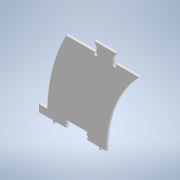
# Autodesk Inventor part: Support C - V2
Saved by Autodesk Inventor 2021 (Build 250183000, 183)
## iProperties
Created: 2020-07-22
Part Number: Support C - V2
Material: Generic
Document SubType Name: Modeling
Designer: Dan Wikman
Density: 1 g/cm^3
Appearance: Default
Author: Dan Wikman
Autodesk Inventor part; units mm, degrees
ref_plane "YZ Plane" through (0, 0, 0) normal (1, 0, 0) x (0, 1, 0)
ref_plane "XZ Plane" through (0, 0, 0) normal (0, 1, 0) x (-1, 0, 0)
ref_plane "XY Plane" through (0, 0, 0) normal (0, 0, 1) x (1, 0, 0)
sketch "Sketch1" plane through (0, 0, 0) normal (0, 0, 1) x (1, 0, 0)
  arc A0 (0, 550) -> (-200, 512.3475) centre (0, 0) ccw construction
  line L0 (-150, -512.4764) -> (-150, -323.4644) construction
  line L1 (-472.3938, -281.6809) -> (-252.3938, -281.6809) construction
  line L2 (-489.0365, 251.6809) -> (-252.3938, 251.6809) construction
  line L3 (-150.0879, 323.2475) -> (-150.0879, 512.2595) construction
  line L4 (-472.3938, 281.6809) -> (-252.3938, 281.6809) construction
  line L5 (-472.3938, -251.6809) -> (-252.3938, -251.6809) construction
  line L6 (-356.435, 15) -> (-576.435, 15) construction
  line L7 (-472.3938, -281.6809) -> (-472.3938, -251.6809) construction
  line L8 (-252.3938, -281.6809) -> (-252.3938, -251.6809) construction
  line L9 (-252.3938, 281.6809) -> (-252.3938, 251.6809) construction
  line L10 (-472.3938, 281.6809) -> (-472.3938, 251.6809) construction
  line L11 (-356.435, 15) -> (-356.435, -15) construction
  line L12 (-356.435, -15) -> (-576.435, -15) construction
  line L13 (-576.435, -15) -> (-576.435, 15) construction
  arc A1 (-0.0879, 356.3469) -> (-150.0879, 323.2475) centre (-0.0879, -0.0881) ccw construction
  arc A2 (-150, -323.4644) -> (-1.4799, -356.5203) centre (-0.0879, -0.0881) ccw construction
  arc A3 (-156.5047, -512.4764) -> (-160, -512.3475) centre (-158.25, -512.3475) ccw construction
  arc A4 (-190, -512.3475) -> (-193.5, -512.3475) centre (-191.75, -512.3475) ccw construction
  line L14 (-178.75, -519.0975) -> (-175, -519.0975) construction
  line L15 (-178.75, -529.0975) -> (-175, -529.0975) construction
  line L16 (-175, -519.0975) -> (-175, -529.0975) construction
  arc A5 (-178.75, -519.0975) -> (-178.75, -522.5975) centre (-178.75, -520.8475) ccw construction
  arc A6 (-178.75, -525.5975) -> (-178.75, -529.0975) centre (-178.75, -527.3475) ccw construction
  line L17 (-171.25, -519.0975) -> (-175, -519.0975) construction
  line L18 (-171.25, -529.0975) -> (-175, -529.0975) construction
  arc A7 (-171.25, -522.5975) -> (-171.25, -519.0975) centre (-171.25, -520.8475) ccw construction
  arc A8 (-171.25, -529.0975) -> (-171.25, -525.5975) centre (-171.25, -527.3475) ccw construction
  line L19 (-252.3938, 251.6809) -> (-489.0365, 251.6809) construction
  arc A9 (-192.6667, 512.3475) -> (-190, 512.3475) centre (-191.3333, 512.3475) ccw construction
  line L20 (-157.3333, 512.3475) -> (-150, 512.3475) construction
  line L21 (-192.6667, 512.3475) -> (-200, 512.3475) construction
  arc A10 (-160, 512.3475) -> (-157.3333, 512.3475) centre (-158.6667, 512.3475) ccw construction
  line L22 (-171.25, 517.8475) -> (-175, 517.8475) construction
  line L23 (-171.25, 520.5142) -> (-171.25, 525.1809) construction
  line L24 (-161.3333, 532.3475) -> (-188.6667, 532.3475) construction
  line L25 (-190, 531.0142) -> (-190, 512.3475) construction
  line L26 (-160, 531.0142) -> (-160, 512.3475) construction
  arc A11 (-160, 531.0142) -> (-161.3333, 532.3475) centre (-161.3333, 531.0142) ccw construction
  arc A12 (-188.6667, 532.3475) -> (-190, 531.0142) centre (-188.6667, 531.0142) ccw construction
  line L27 (-171.25, 527.8475) -> (-175, 527.8475) construction
  line L28 (-175, 532.3475) -> (-175, 535.9358) construction
  line L29 (-175, 517.8475) -> (-175, 527.8475) construction
  arc A13 (-171.25, 517.8475) -> (-171.25, 520.5142) centre (-171.25, 519.1809) ccw construction
  arc A14 (-171.25, 525.1809) -> (-171.25, 527.8475) centre (-171.25, 526.5142) ccw construction
  line L30 (-178.75, 517.8475) -> (-175, 517.8475) construction
  arc A15 (-178.75, 520.5142) -> (-178.75, 517.8475) centre (-178.75, 519.1809) ccw construction
  line L31 (-178.75, 520.5142) -> (-178.75, 525.1809) construction
  arc A16 (-178.75, 527.8475) -> (-178.75, 525.1809) centre (-178.75, 526.5142) ccw construction
  line L32 (-178.75, 527.8475) -> (-175, 527.8475) construction
  arc A17 (-334.9122, -265.623) -> (-335.582, -268.123) centre (-330.582, -268.123) ccw construction
  line L33 (-328.3782, -254.3059) -> (-334.9122, -265.623) construction
  arc A18 (-328.3782, -254.3059) -> (-329.8938, -251.6809) centre (-329.8938, -253.4309) ccw construction
  line L34 (-329.8938, -251.6809) -> (-394.8938, -251.6809) construction
  line L35 (-362.3938, -251.6809) -> (-362.3938, -293.6041) construction
  arc A19 (-389.2055, -268.123) -> (-389.8754, -265.623) centre (-394.2055, -268.123) ccw construction
  arc A20 (-394.8938, -251.6809) -> (-396.4093, -254.3059) centre (-394.8938, -253.4309) ccw construction
  line L36 (-396.4093, -254.3059) -> (-389.8754, -265.623) construction
  arc A21 (-389.2055, -291.6809) -> (-389.2055, -288.1809) centre (-389.2055, -289.9309) ccw construction
  line L37 (-389.2055, -291.6809) -> (-396.7055, -291.6809) construction
  line L38 (-396.7055, -281.6809) -> (-472.3938, -281.6809) construction
  line L39 (-328.082, -281.6809) -> (-252.3938, -281.6809) construction
  line L40 (-252.4816, -287.4356) -> (-210.9842, -287.4356) construction
  arc A22 (-150.0879, 323.2475) -> (-250.6303, 253.4358) centre (-0.0879, -0.0881) ccw construction
  arc A23 (-210.9842, -287.4356) -> (-150, -323.4644) centre (-0.0879, -0.0881) ccw construction
  arc A24 (-200, 512.3475) -> (-491.4496, 246.9358) centre (0, 0) ccw construction
  arc A25 (-472.3938, -281.6809) -> (-246.475, -491.6809) centre (0, 0) ccw construction
  line L41 (-171.25, -436.2204) -> (-171.25, -399.7204) construction
  line L42 (-178.75, -436.2204) -> (-178.75, -399.7204) construction
  line L43 (-177, -437.9704) -> (-173, -437.9704) construction
  line L44 (-177, -397.9704) -> (-173, -397.9704) construction
  arc A26 (-177, -397.9704) -> (-178.75, -399.7204) centre (-177, -399.7204) ccw construction
  arc A27 (-178.75, -436.2204) -> (-177, -437.9704) centre (-177, -436.2204) ccw construction
  arc A28 (-173, -437.9704) -> (-171.25, -436.2204) centre (-173, -436.2204) ccw construction
  arc A29 (-171.25, -399.7204) -> (-173, -397.9704) centre (-173, -399.7204) ccw construction
  line L45 (-200, -512.3475) -> (-200, -491.6809) construction
  arc A30 (-200, -491.6809) -> (-203.5, -491.6809) centre (-201.75, -491.6809) ccw construction
  line L46 (-160, -512.3475) -> (-160, -532.5975) construction
  line L47 (-161.75, -534.3475) -> (-188.25, -534.3475) construction
  line L48 (-190, -532.5975) -> (-190, -512.3475) construction
  line L49 (-171.25, -522.5975) -> (-171.25, -525.5975) construction
  line L50 (-178.75, -522.5975) -> (-178.75, -525.5975) construction
  arc A31 (-190, -532.5975) -> (-188.25, -534.3475) centre (-188.25, -532.5975) ccw construction
  arc A32 (-161.75, -534.3475) -> (-160, -532.5975) centre (-161.75, -532.5975) ccw construction
  line L51 (-156.5047, -512.4764) -> (-150, -512.4764) construction
  line L52 (-193.5, -512.3475) -> (-200, -512.3475) construction
  line L53 (-203.5, -491.6809) -> (-246.475, -491.6809) construction
  arc A33 (-396.7055, -288.1809) -> (-396.7055, -291.6809) centre (-396.7055, -289.9309) ccw construction
  line L54 (-396.7055, -281.6809) -> (-396.7055, -288.1809) construction
  line L55 (-389.2055, -288.1809) -> (-389.2055, -268.123) construction
  arc A34 (-335.582, -288.1809) -> (-335.582, -291.6809) centre (-335.582, -289.9309) ccw construction
  line L56 (-335.582, -291.6809) -> (-328.082, -291.6809) construction
  arc A35 (-328.082, -291.6809) -> (-328.082, -288.1809) centre (-328.082, -289.9309) ccw construction
  line L57 (-328.082, -281.6809) -> (-328.082, -288.1809) construction
  line L58 (-335.582, -288.1809) -> (-335.582, -268.123) construction
  arc A36 (-252.3938, -283.9378) -> (-252.4816, -287.4356) centre (-252.4816, -285.6856) ccw construction
  line L59 (-252.3938, -283.9378) -> (-252.3938, -281.6809) construction
  arc A37 (-479.7691, -25) -> (-479.7691, -21.5) centre (-479.7691, -23.25) ccw construction
  arc A38 (-479.7691, -1.4421) -> (-480.4389, 1.0579) centre (-484.7691, -1.4421) ccw construction
  line L60 (-486.9729, 12.375) -> (-480.4389, 1.0579) construction
  arc A39 (-485.4573, 15) -> (-486.9729, 12.375) centre (-485.4573, 13.25) ccw construction
  line L61 (-420.4573, 15) -> (-485.4573, 15) construction
  arc A40 (-425.4757, 1.0579) -> (-426.1456, -1.4421) centre (-421.1456, -1.4421) ccw construction
  arc A41 (-418.9418, 12.375) -> (-420.4573, 15) centre (-420.4573, 13.25) ccw construction
  line L62 (-418.9418, 12.375) -> (-425.4757, 1.0579) construction
  line L63 (-452.9573, 15) -> (-452.9573, -26.9232) construction
  line L64 (-479.7691, -25) -> (-487.2691, -25) construction
  line L65 (-487.2691, -15) -> (-549.7954, -15) construction
  arc A42 (-487.2691, -21.5) -> (-487.2691, -25) centre (-487.2691, -23.25) ccw construction
  line L66 (-487.2691, -15) -> (-487.2691, -21.5) construction
  line L67 (-479.7691, -21.5) -> (-479.7691, -1.4421) construction
  line L68 (-426.1456, -21.5) -> (-426.1456, -1.4421) construction
  arc A43 (-426.1456, -21.5) -> (-426.1456, -25) centre (-426.1456, -23.25) ccw construction
  line L69 (-426.1456, -25) -> (-418.6456, -25) construction
  arc A44 (-418.6456, -25) -> (-418.6456, -21.5) centre (-418.6456, -23.25) ccw construction
  line L70 (-418.6456, -15) -> (-418.6456, -21.5) construction
  line L71 (276.2049, -135.3556) -> (280.6774, -127.609)
  line L72 (279.2083, -124.984) -> (246.5502, -124.984)
  arc A45 (319.0505, -151.484) -> (319.0505, -147.984) centre (319.0505, -149.734) ccw
  arc A46 (328.5505, -147.9841) -> (325.0505, -147.9841) centre (326.8005, -147.9841) ccw
  line L73 (319.0505, -147.984) -> (280.8619, -147.984)
  arc A47 (214.0502, -164.7817) -> (212.5346, -167.4067) centre (214.0502, -166.5317) ccw
  arc A48 (280.5657, -167.4067) -> (279.0502, -164.7817) centre (279.0502, -166.5317) ccw
  arc A49 (274.0318, -178.7238) -> (273.3619, -181.2238) centre (278.3619, -181.2238) ccw
  line L74 (280.5657, -167.4067) -> (274.0318, -178.7238)
  line L75 (273.3619, -201.2817) -> (273.3619, -181.2238)
  arc A50 (273.3619, -201.2817) -> (273.3619, -204.7817) centre (273.3619, -203.0317) ccw
  line L76 (273.3619, -204.7817) -> (280.8619, -204.7817)
  arc A51 (280.8619, -204.7817) -> (280.8619, -201.2817) centre (280.8619, -203.0317) ccw
  line L77 (280.8619, -194.7817) -> (280.8619, -201.2817)
  line L78 (212.2384, -194.7817) -> (212.2384, -201.2817)
  arc A52 (212.2384, -201.2817) -> (212.2384, -204.7817) centre (212.2384, -203.0317) ccw
  arc A53 (219.7384, -204.7817) -> (219.7384, -201.2817) centre (219.7384, -203.0317) ccw
  line L79 (279.0502, -164.7817) -> (214.0502, -164.7817)
  line L80 (219.7384, -201.2817) -> (219.7384, -181.2238)
  line L81 (219.7384, -204.7817) -> (212.2384, -204.7817)
  arc A54 (219.7384, -181.2238) -> (219.0686, -178.7238) centre (214.7384, -181.2238) ccw
  line L82 (212.5346, -167.4067) -> (219.0686, -178.7238)
  line L83 (212.2384, -194.7817) -> (136.5502, -194.7817)
  line L84 (280.8619, -194.7817) -> (356.5502, -194.7817)
  line L85 (325.0505, -147.9841) -> (325.0505, -154.9841)
  line L86 (325.0505, -154.9841) -> (319.0505, -154.9841)
  line L87 (319.0505, -151.484) -> (319.0505, -154.9841)
  line L88 (246.5502, -124.984) -> (246.5502, -110.6064)
  arc A55 (280.6774, -127.609) -> (279.2083, -124.984) centre (279.1622, -126.7334) ccw
  arc A56 (280.8619, -138.8556) -> (280.8619, -135.3556) centre (280.8619, -137.1056) ccw
  line L89 (276.2049, -135.3556) -> (280.8619, -135.3556)
  line L90 (246.5502, -164.7817) -> (246.5502, -170.2759)
  line L91 (280.8619, -147.984) -> (280.8619, -138.8556)
  arc A57 (168.0499, -147.9841) -> (164.5499, -147.9841) centre (166.2999, -147.9841) ccw
  arc A58 (174.0499, -147.984) -> (174.0499, -151.484) centre (174.0499, -149.734) ccw
  line L92 (213.8921, -124.984) -> (246.5502, -124.984)
  line L93 (174.0499, -147.984) -> (212.2384, -147.984)
  line L94 (216.8955, -135.3556) -> (212.423, -127.609)
  line L95 (168.0499, -147.9841) -> (168.0499, -154.9841)
  line L96 (168.0499, -154.9841) -> (174.0499, -154.9841)
  line L97 (174.0499, -151.484) -> (174.0499, -154.9841)
  arc A59 (213.8921, -124.984) -> (212.423, -127.609) centre (213.9382, -126.7334) ccw
  arc A60 (212.2384, -135.3556) -> (212.2384, -138.8556) centre (212.2384, -137.1056) ccw
  line L98 (216.8955, -135.3556) -> (212.2384, -135.3556)
  line L99 (212.2384, -147.984) -> (212.2384, -138.8556)
  arc A61 (-280.4036, -274.8689) -> (-283.8935, -274.681) centre (-282.1435, -274.681) ccw construction
  arc A62 (-289.8935, -278.1809) -> (-289.8935, -274.6809) centre (-289.8935, -276.4309) ccw construction
  line L100 (-329.7357, -251.6809) -> (-362.3938, -251.6809) construction
  line L101 (-289.8935, -274.6809) -> (-328.082, -274.6809) construction
  line L102 (-332.7391, -262.0525) -> (-328.2666, -254.3059) construction
  line L103 (-283.8935, -274.681) -> (-283.8935, -281.681) construction
  line L104 (-283.8935, -281.681) -> (-289.8935, -281.681) construction
  line L105 (-289.8935, -278.1809) -> (-289.8935, -281.681) construction
  arc A63 (-328.2666, -254.3059) -> (-329.7357, -251.6809) centre (-329.7818, -253.4303) ccw construction
  arc A64 (-328.082, -265.5525) -> (-328.082, -262.0525) centre (-328.082, -263.8025) ccw construction
  line L106 (-332.7391, -262.0525) -> (-328.082, -262.0525) construction
  line L107 (-328.082, -274.6809) -> (-328.082, -265.5525) construction
  line L108 (-392.0485, -262.0525) -> (-396.7055, -262.0525) construction
  arc A65 (-396.7055, -262.0525) -> (-396.7055, -265.5525) centre (-396.7055, -263.8025) ccw construction
  line L109 (-392.0485, -262.0525) -> (-396.521, -254.3059) construction
  arc A66 (-395.0519, -251.6809) -> (-396.521, -254.3059) centre (-395.0058, -253.4303) ccw construction
  line L110 (-396.7055, -274.6809) -> (-396.7055, -265.5525) construction
  line L111 (-434.8941, -278.1809) -> (-434.8941, -281.681) construction
  line L112 (-434.8941, -274.6809) -> (-396.7055, -274.6809) construction
  arc A67 (-434.8941, -274.6809) -> (-434.8941, -278.1809) centre (-434.8941, -276.4309) ccw construction
  line L113 (-440.8941, -281.681) -> (-434.8941, -281.681) construction
  line L114 (-440.8941, -274.681) -> (-440.8941, -281.681) construction
  arc A68 (-440.8941, -274.681) -> (-444.3912, -274.7808) centre (-442.6441, -274.681) ccw construction
  line L115 (-395.0519, -251.6809) -> (-362.3938, -251.6809) construction
  line L116 (-444.3912, -274.7808) -> (-476.4404, -274.7808) construction
  arc A69 (-355.8791, -21.5) -> (-227.1151, -274.8689) centre (-0.0879, -0.0881) ccw construction
  arc A70 (-549.7954, -15) -> (-476.4404, -274.7808) centre (0, 0) ccw construction
  line L117 (-280.4036, -274.8689) -> (-227.1151, -274.8689) construction
  line L118 (-364.1192, -15) -> (-364.1192, -18) construction
  arc A71 (-364.1192, -18) -> (-364.1192, -21.5) centre (-364.1192, -19.75) ccw construction
  line L119 (-364.1192, -21.5) -> (-355.8791, -21.5) construction
  line L120 (-356.1192, -15) -> (-356.435, -15) construction
  line L121 (-364.1192, -15) -> (-549.7954, -15) construction
  line L122 (-418.6456, -15) -> (-364.1192, -15) construction
  arc A72 (-370.957, -8.0002) -> (-374.457, -8.0002) centre (-372.707, -8.0002) ccw
  arc A73 (-380.457, -11.5) -> (-380.457, -8) centre (-380.457, -9.75) ccw
  line L123 (-420.2992, 15) -> (-452.9573, 15)
  line L124 (-380.457, -8) -> (-418.6456, -8)
  line L125 (-423.3026, 4.6284) -> (-418.8301, 12.375)
  line L126 (-374.457, -8.0002) -> (-374.457, -15.0002)
  line L127 (-374.457, -15.0002) -> (-380.457, -15.0002)
  line L128 (-380.457, -11.5) -> (-380.457, -15.0002)
  line L129 (-452.9573, 15) -> (-452.9573, 29.3776)
  arc A74 (-418.8301, 12.375) -> (-420.2992, 15) centre (-420.3453, 13.2506) ccw
  arc A75 (-418.6456, 1.1284) -> (-418.6456, 4.6284) centre (-418.6456, 2.8784) ccw
  line L130 (-423.3026, 4.6284) -> (-418.6456, 4.6284)
  line L131 (-418.6456, -8) -> (-418.6456, 1.1284)
  line L132 (-482.612, 4.6284) -> (-487.2691, 4.6284)
  arc A76 (-487.2691, 4.6284) -> (-487.2691, 1.1284) centre (-487.2691, 2.8784) ccw
  line L133 (-482.612, 4.6284) -> (-487.0845, 12.375)
  arc A77 (-485.6154, 15) -> (-487.0845, 12.375) centre (-485.5693, 13.2506) ccw
  line L134 (-487.2691, -8) -> (-487.2691, 1.1284)
  line L135 (-525.4576, -11.5) -> (-525.4576, -15.0002)
  line L136 (-525.4576, -8) -> (-487.2691, -8)
  arc A78 (-525.4576, -8) -> (-525.4576, -11.5) centre (-525.4576, -9.75) ccw
  line L137 (-531.4576, -15.0002) -> (-525.4576, -15.0002)
  line L138 (-531.4576, -8.0002) -> (-531.4576, -15.0002)
  arc A79 (-531.4576, -8.0002) -> (-534.9576, -8.0002) centre (-533.2076, -8.0002) ccw
  line L139 (-485.6154, 15) -> (-452.9573, 15)
  line L140 (-370.957, -8.0002) -> (-356.435, -8.0002)
  line L141 (-534.9576, -8.0002) -> (-549.9418, -8.0002)
  line L142 (-395.8328, 253.4358) -> (-471.4936, 253.4358)
  arc A80 (-488.1712, 253.3553) -> (-549.7954, 15) centre (0, 0) ccw
  line L143 (-549.7954, 15) -> (-576.435, 15)
  line L144 (-576.435, 15) -> (-576.435, -8.0002)
  line L145 (-549.9418, -8.0002) -> (-576.435, -8.0002)
  line L146 (-356.435, 15) -> (-356.435, -8.0002)
  line L147 (-356.435, 15) -> (-356.2033, 15)
  arc A81 (-251.4953, 252.5781) -> (-356.2033, 15) centre (-0.0879, -0.0881) ccw
  arc A82 (-356.435, 7.824) -> (-356.435, -8.0002) centre (-0.0879, -0.0881) ccw
  arc A83 (-250.6303, 253.4358) -> (-251.4953, 252.5781) centre (-0.0879, -0.0881) ccw
  line L148 (-327.2093, 253.4358) -> (-327.2093, 246.9358)
  arc A84 (-327.2093, 243.4358) -> (-327.2093, 246.9358) centre (-327.2093, 245.1858) ccw
  line L149 (-395.8328, 253.4358) -> (-395.8328, 246.9358)
  arc A85 (-395.8328, 246.9358) -> (-395.8328, 243.4358) centre (-395.8328, 245.1858) ccw
  arc A86 (-388.3328, 243.4358) -> (-388.3328, 246.9358) centre (-388.3328, 245.1858) ccw
  line L150 (-388.3328, 246.9358) -> (-388.3328, 266.9938)
  line L151 (-388.3328, 243.4358) -> (-395.8328, 243.4358)
  arc A87 (-388.3328, 266.9938) -> (-389.0027, 269.4938) centre (-393.3328, 266.9938) ccw
  line L152 (-395.5366, 280.8108) -> (-389.0027, 269.4938)
  arc A88 (-394.021, 283.4358) -> (-395.5366, 280.8108) centre (-394.021, 281.6858) ccw
  line L153 (-329.021, 283.4358) -> (-394.021, 283.4358)
  arc A89 (-334.0394, 269.4938) -> (-334.7093, 266.9938) centre (-329.7093, 266.9938) ccw
  arc A90 (-327.5055, 280.8108) -> (-329.021, 283.4358) centre (-329.021, 281.6858) ccw
  line L154 (-327.5055, 280.8108) -> (-334.0394, 269.4938)
  arc A91 (-334.7093, 246.9358) -> (-334.7093, 243.4358) centre (-334.7093, 245.1858) ccw
  line L155 (-334.7093, 243.4358) -> (-327.2093, 243.4358)
  line L156 (-334.7093, 246.9358) -> (-334.7093, 266.9938)
  line L157 (-361.521, 283.4358) -> (-361.521, 277.9417)
  line L158 (-327.2093, 253.4358) -> (-250.6303, 253.4358)
  line L159 (-251.4953, 253.4358) -> (-251.4953, 252.5781)
  line L160 (-471.4936, 253.3553) -> (-488.1712, 253.3553)
  line L161 (-471.4936, 253.4358) -> (-471.4936, 253.3553)
  line L162 (-471.4936, 251.6809) -> (-471.4936, 250.4358)
  point P0 (0, 512.3475)
  point P1 (0, -512.3475)
  point P2 (0, 0)
  point P3 (-190, -534.3475)
  point P4 (-160, -534.3475)
  point P5 (-59.9119, -534.1417)
  point P6 (-160, 532.3475)
  point P7 (-190, 532.3475)
  point P8 (-389.2055, -259.0142)
  point P9 (-479.7691, 7.6667)
  point P10 (328.5476, -148.0839)
  point P11 (328.0311, -152.0673)
  point P12 (329.3645, -149.3173)
  point P13 (219.7384, -172.1151)
  point P14 (164.5527, -148.0839)
  point P15 (165.0692, -152.0673)
  point P16 (163.7359, -149.3173)
  point P17 (-280.9128, -278.7642)
  point P18 (-279.5795, -276.0142)
  point P19 (-443.8747, -278.7642)
  point P20 (-445.2081, -276.0142)
  point P21 (-370.9599, -8.1)
  point P22 (-371.4764, -12.0833)
  point P23 (-370.143, -9.3333)
  point P24 (-534.4382, -12.0833)
  point P25 (-534.9548, -8.1)
  point P26 (-535.7716, -9.3333)
  point P27 (-388.3328, 276.1025)
  dimension "d13" = 550
  dimension "d17" = 200
  dimension "d18" = 0
  dimension "d19" = 150
  dimension "d54" = 220
  dimension "d56" = 220
  dimension "d57" = 30
  dimension "d73" = 236.6809
  dimension "d74" = 236.6809
  dimension "d75" = 576.435
  dimension "d76" = 472.3938
  dimension "d77" = 472.3938
  dimension "d78" = 30
  dimension "d81" = 220
  dimension "d82" = 252.3938
  dimension "d85" = 356.435
  dimension "d88" = 3.5
  dimension "d89" = 30
  dimension "d90" = 22
  dimension "d91" = 3.5
  dimension "d103" = 3.75
  dimension "d104" = 3.75
  dimension "d105" = 2.6667
  dimension "d106" = 30
  dimension "d107" = 20
  dimension "d108" = 2.6667
  dimension "d109" = 1.3333
  dimension "d110" = 7.3333
  dimension "d111" = 7.3333
  dimension "d112" = 7.5
  dimension "d113" = 3.75
  dimension "d114" = 3.75
  dimension "d134" = 3.5
  dimension "d135" = 65
  dimension "d136" = 65
  dimension "d137" = 7.3333
  dimension "d138" = 60
  dimension "d139" = 5
  dimension "d140" = 7.5
  dimension "d148" = 1.75
  dimension "d151" = 40
  dimension "d152" = 74.506
  dimension "d153" = 20.6667
  dimension "d154" = 3.5
  dimension "d155" = 189.012
  dimension "d159" = 1.75
  dimension "d160" = 1.75
  dimension "d161" = 1.75
  dimension "d164" = 7.5
  dimension "d168" = 21.25
  dimension "d170" = 30
  dimension "d171" = 1.75
  dimension "d172" = 10
  dimension "d173" = 3.5
  dimension "d177" = 3.5
  dimension "d178" = 65
  dimension "d179" = 65
  dimension "d180" = 7.3333
  dimension "d181" = 60
  dimension "d182" = 5
  dimension "d183" = 7.5
  dimension "d185" = 1.75
  dimension "d186" = 10
  dimension "d192" = 1.75
  constraints: 326 end point, 194 point on circle, 92 centre point, 72 symmetric about line, 30 tangent, 30 vertical, 23 horizontal, 15 perpendicular, 15 point on line, 5 midpoint, 4 equal radius, 3 collinear, 2 parallel, 1 coincident, 29 other
  measures "d13" radius of A0
  measures "d17" distance of point (0, 512.348) A0.end
  measures "d18" horizontal distance of point (0, 0) point (0, 512.348)
  measures "d19" distance from line of point (0, 0) L0
  measures "d54" distance of L6.start L6.end
  measures "d56" distance of L1.start L1.end
  measures "d57" distance of L1.end L5.end
  measures "d73" distance between parallel lines of L5 L12
  measures "d74" distance between parallel lines of L2 L6
  measures "d75" distance from line of L13 point (0, 0)
  measures "d76" distance from line of point (0, 0) L7
  measures "d77" distance from line of point (0, 0) L10
  measures "d78" distance of L6.start L11.end
  measures "d81" distance between parallel lines of L9 L10
  measures "d82" distance from line of point (0, 0) L9
  measures "d85" distance from line of A0.centre L11
  measures "d88" diameter of A3
  measures "d89" distance of point (-190, -534.348) point (-160, -534.348)
  measures "d90" distance of point (-160, -534.348) L46.start
  measures "d91" diameter of A4
  measures "d103" distance of L14.start L14.end
  measures "d104" distance of L15.start L15.end
  measures "d105" diameter of A9
  measures "d106" distance of point (-160, 532.348) point (-190, 532.348)
  measures "d107" distance of point (-190, 532.348) L25.end
  measures "d108" diameter of A10
  measures "d109" radius of A11
  measures "d110" distance of L20.start L20.end
  measures "d111" distance of L21.start L21.end
  measures "d112" diameter of L23 L29
  measures "d113" distance of L22.start L22.end
  measures "d114" distance of L27.start L27.end
  measures "d134" diameter of A18
  measures "d135" distance of L34.start L34.end
  measures "d136" distance between centres of A18 A20
  measures "d137" distance from line of point (-389.206, -259.014) L34
  measures "d138" angle of L34 L36
  measures "d139" radius of A19
  measures "d140" distance of L37.start L37.end
  measures "d148" radius of A26
  measures "d151" distance between parallel lines of L43 L44
  measures "d152" distance from line of L0.end L44
  measures "d153" distance of L45.start L45.end
  measures "d154" diameter of A30
  measures "d155" distance of L0.start L0.end
  measures "d159" radius of A5
  measures "d160" radius of A8
  measures "d161" radius of A31
  measures "d164" distance between parallel lines of L42 L41
  measures "d168" distance between parallel lines of L41 L0
  measures "d170" distance between parallel lines of L39 L34
  measures "d171" radius of A21
  measures "d172" distance between parallel lines of L38 L37
  measures "d173" diameter of A36
  measures "d177" diameter of A41
  measures "d178" distance of L61.start L61.end
  measures "d179" distance between centres of A41 A39
  measures "d180" distance from line of point (-479.769, 7.667) L61
  measures "d181" angle of L61 L60
  measures "d182" radius of A38
  measures "d183" distance of L64.start L64.end
  measures "d185" radius of A37
  measures "d186" distance between parallel lines of L65 L64
  measures "d192" radius of A45
extrude "Extrusion3" add sketch "Sketch1" along normal blind 7 contours A72 L126 L127 L128 A73 L124 L131 A75 L130 L125 A74 L123 L139 A77 L133 L132 A76 L134 L136 A78 L135 L137 L138 A79 L141 L145 L144 L143 A80 L160 L161 L142 L149 A85 L151 A86 L150 A87 L152 A88 L153 A90 L154 A89 L156 A91 L155 A84 L148 L158 L159 A81 L147 L146 A82 L140 | A82 L146
body "Solid3"
